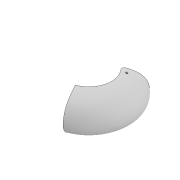
# Autodesk Inventor part: Spline_cover_p2
Saved by Autodesk Inventor 2022 (Build 260153000, 153)
## iProperties
Created: 2022-08-08
Part Number: Spline_cover_p2
Material: Generic
Document SubType Name: Modeling
Designer: dell
Density: 1 g/cm^3
Appearance: Default
Author: dell
Autodesk Inventor part; units mm, degrees
ref_plane "YZ Plane" through (0, 0, 0) normal (1, 0, 0) x (0, 1, 0)
ref_plane "XY Plane" through (0, 0, 0) normal (0, 0, 1) x (1, 0, 0)
sketch "Sketch1" plane through (0, 0, 0) normal (1, 0, 0) x (0, 1, 0)
  line L0 (0, 0) -> (40, 0) construction
  line L1 (40, 0) -> (40, -45) construction
  line L2 (40, -45) -> (0, -45) construction
  line L3 (0, -45) -> (0, 0) construction
  line L4 (40, 0) -> (40, -9.142735) construction
  line L5 (40, -9.142735) -> (38.525963, -21.237022) construction
  line L6 (38.525963, -21.237022) -> (35.297324, -29.785022) construction
  line L7 (35.297324, -29.785022) -> (30.699911, -38.62494) construction
  line L8 (30.699911, -38.62494) -> (23.434277, -45) construction
  line L9 (23.434277, -45) -> (12.360751, -46.153187) construction
  line L10 (12.360751, -46.153187) -> (6.865194, -41.708799) construction
  line L11 (6.865194, -41.708799) -> (2, -33.241369) construction
  line L12 (2, -33.241369) -> (0, -21.237022) construction
  line L13 (0, -21.237022) -> (0, -7.673177) construction
  line L14 (0, -7.673177) -> (0, 0) construction
  spline S0 degree 4 poles (40, 0) (40, -9.142735) (38.525963, -21.237022) (35.297324, -29.785022) (30.699911, -38.62494) (23.434277, -45) (12.360751, -46.153187) (6.865194, -41.708799) (2, -33.241369) (0, -21.237022) (0, -7.673177) (0, 0) knots 1 1 1 1 1 2 3 4 5 6 7 8 9 9 9 9 9
  line L15 (40, 0) -> (38, 0)
  line L16 (2, 0) -> (0, 0)
  line L17 (-27.078772, 0) -> (60.134312, 0)
  spline S1 degree 5 poles (38, 0) (38.00002, -3.295699) (37.908895, -6.591804) (37.706159, -9.883511) (37.15964, -15.041818) (36.122223, -20.11749) (35.672397, -21.947111) (34.753942, -25.041621) (33.576541, -28.044982) (33.042006, -29.277194) (31.973625, -31.539109) (30.754186, -33.723013) (30.151816, -34.7132) (28.902483, -36.553417) (27.448407, -38.235325) (26.700243, -38.994334) (25.099157, -40.385486) (23.284756, -41.483929) (22.333846, -41.945771) (20.386186, -42.692204) (18.341418, -43.108773) (17.31796, -43.233233) (15.464811, -43.309782) (13.636071, -43.032229) (12.837366, -42.829752) (11.316297, -42.203147) (10.017419, -41.196433) (9.430689, -40.62686) (8.174127, -39.209264) (7.138797, -37.618902) (6.604619, -36.681361) (5.454914, -34.371466) (4.585956, -31.939668) (4.162526, -30.498793) (3.276062, -26.856965) (2.745197, -23.142919) (2.520562, -20.90664) (2.129588, -15.387668) (2.020977, -9.855061) (1.999807, -6.570322) (2.000037, -3.285078) (2, 0) knots 0 0 0 0 0 0 0.1603328 0.1603328 0.1603328 0.2518749 0.2518749 0.2518749 0.3171681 0.3171681 0.3171681 0.373494 0.373494 0.373494 0.42516635 0.42516635 0.42516635 0.47629827 0.47629827 0.47629827 0.52631034 0.52631034 0.52631034 0.56599365 0.56599365 0.56599365 0.60556263 0.60556263 0.60556263 0.65797827 0.65797827 0.65797827 0.73090825 0.73090825 0.73090825 0.84018584 0.84018584 0.84018584 1 1 1 1 1 1
  dimension "d4" = 2
  dimension "d2" = 45
  dimension "d3" = 40
  constraints: 12 end point, 4 point on line, 2 collinear, 2 parallel, 1 coincident, 1 horizontal, 1 horizontal alignment, 1 perpendicular, 5 other
  measures "d2" distance between parallel lines of L0 L2
  measures "d3" distance between parallel lines of L1 L3
revolve "Revolution1" add sketch "Sketch1" angle 160 about axis through (0, -10, 0) along (0, -1, 0) contours S0 L16 S1 L15
thicken "Thicken1" operation add thickness 2.3 both sides no extend neighbours yes toward (0.223087, 0.8949463, -0.386398) faces at (15.97026, 33.96398, -27.661302)
thicken "Thicken2" operation add thickness 2.3 both sides no extend neighbours yes toward (0.1018286, -0.9911257, 0.0854443) faces at (18.315686, 2.89993, 15.368686)
sketch "Sketch2" plane through (0, 0, 0) normal (0, 1, 0) x (-1, 0, 0)
  circle A0 centre (0, 0) radius 15
  dimension "d6" = 30
  constraints: 1 centre point, 1 coincident
  measures "d6" diameter of A0
extrude "Extrusion1" cut sketch "Sketch2" along normal mid plane 20
sketch "Sketch3" plane through (0, 0, 0) normal (0, 1, 0) x (-1, 0, 0)
  circle A0 centre (-23.6, -4.5) radius 1.05
  circle A1 centre (-23.6, -18) radius 1.05
  point P0 (0, 0)
  dimension "d9" = 2.1
  dimension "d10" = 2.1
  dimension "d12" = 4.5
  dimension "d14" = 18
  dimension "d54" = 23.6
  dimension "d55" = 23.6
  constraints: 2 centre point
  measures "d9" diameter of A0
  measures "d10" diameter of A1
  measures "d12" vertical distance of point (0, 0) A0.centre
  measures "d14" vertical distance of point (0, 0) A1.centre
  measures "d54" horizontal distance of point (0, 0) A1.centre
  measures "d55" horizontal distance of point (0, 0) A0.centre
extrude "Extrusion2" cut sketch "Sketch3" along normal mid plane 100
sketch "Sketch4" plane through (0, 0, 0) normal (0, 1, 0) x (-1, 0, 0)
  line L0 (-5.130302, 14.095389) -> (0, 0)
  line L1 (0, -15) -> (0, 0)
  line L2 (0, 0) -> (-47.15263, -56.194317)
  line L3 (0, -67.024453) -> (0, 27.980921)
  line L4 (-47.15263, -56.194317) -> (0, -56.194317)
  point P0 (0, -20)
  dimension "d56" = 40
  constraints: 4 end point, 1 perpendicular, 1 point on line, 4 other
  measures "d56" angle of L3 L2
extrude "Extrusion3" cut sketch "Sketch4" along normal mid plane 100
ref_plane "Work Plane2" through (0, 30, 0) normal (0, 1, 0) x (-1, 0, 0)
sketch "Sketch8" plane through (0, 30, 0) normal (0, 1, 0) x (-1, 0, 0)
  circle A0 centre (0, 0) radius 25
  dimension "d39" = 50
  constraints: 1 centre point, 1 coincident
  measures "d39" diameter of A0
extrude "Extrusion7" cut sketch "Sketch8" along normal blind 20
ref_plane "Work Plane4" through (0, 1.7, 0) normal (0, 1, 0) x (-1, 0, 0)
sketch "Sketch10" plane through (0, 1.7, 0) normal (0, 1, 0) x (-1, 0, 0)
  spline S0 degree 8 poles (-9.641814, -11.490667) (-10.644411, -10.649388) (-11.563523, -9.707792) (-12.386777, -8.67602) (-13.104089, -7.565649) (-13.707043, -6.389254) (-14.188956, -5.160408) (-14.544846, -3.893636) (-14.999386, -1.315809) (-15.098221, -0.003711) (-15.06566, 1.31585) (-14.90142, 2.627522) (-14.607137, 3.916265) (-14.186418, 5.167383) (-13.64478, 6.366549) (-12.335983, 8.633451) (-11.568294, 9.702107) (-10.695154, 10.692019) (-9.726211, 11.591247) (-8.672389, 12.38932) (-7.545897, 13.077298) (-6.360169, 13.647754) (-5.130302, 14.095389) knots 0 0 0 0 0 0 0 0 0 0.33333333 0.33333333 0.33333333 0.33333333 0.33333333 0.33333333 0.33333333 0.66666667 0.66666667 0.66666667 0.66666667 0.66666667 0.66666667 0.66666667 1 1 1 1 1 1 1 1 1
  line L0 (-9.641814, -11.490667) -> (-11.570177, -13.7888)
  line L1 (-6.156363, 16.914467) -> (-5.130302, 14.095389)
  spline S1 degree 5 poles (-11.570177, -13.7888) (-14.457845, -11.365394) (-16.712631, -8.186826) (-18.06443, -4.470984) (-18.697883, 3.296941) (-15.445845, 10.37975) (-12.904677, 13.409156) (-9.698737, 15.624851) (-6.156363, 16.914467) knots 0 0 0 0 0 0 0.5 0.5 0.5 1 1 1 1 1 1
  point P0 (0, 0)
  dimension "d51" = 3
  constraints: 4 end point, 4 other
extrude "Extrusion9" add sketch "Sketch10" against normal blind 3
chamfer "Chamfer3" distance 1 angle 45 1 edges at (15.5377, 14.3189, 42.6894)
fillet "Fillet1" radius 5 1 edges at (16.0697, 38.1647, -19.1511)
body "Solid1"
